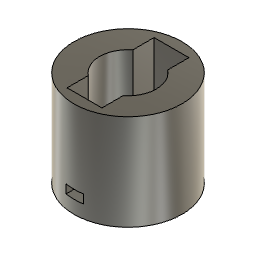
_Button housing.67708ecc-d906-4079-a98f-9e7625d90127 (Autodesk Fusion 360 design; units mm, degrees)
Autodesk Fusion 360 part; units mm, degrees
sketch "Sketch1" plane through (0, 0, 0) normal (0, 0, 1) x (1, 0, 0)
  circle A0 centre (0, 0) radius 31
  dimension "d1" = 62
  constraint coincident A0.centre origin
  measures "d1" diameter of A0
extrude "Extrude1" add sketch "Sketch1" along normal blind 55
sketch "Sketch2" plane through (0, 0, 55) normal (0, 0, 1) x (-1, 0, 0)
  circle A0 centre (0, 0) radius 31
  circle A1 centre (0, 0) radius 16.25
  dimension "d4" = 32.5
  constraint coincident A0.centre A1.centre
  measures "d4" diameter of A1
extrude "Extrude2" cut sketch "Sketch2" against normal blind 50 contours A1
sketch "Sketch3" plane through (0, 0, 55) normal (0, 0, 1) x (-1, 0, 0)
  circle A0 centre (0, 0) radius 16.25
  circle A1 centre (0, 0) radius 31
  line L0 (10, -25) -> (-10, -25)
  line L1 (-10, -25) -> (-10, 25)
  line L2 (-10, 25) -> (10, 25)
  line L3 (10, 25) -> (10, -25)
  line L4 (10, -25) -> (-10, 25) construction
  line L5 (-10, -25) -> (10, 25) construction
  dimension "d7" = 20
  dimension "d8" = 50
  constraint horizontal L0
  constraint perpendicular L0 L1
  constraint parallel L0 L2
  constraint parallel L1 L3
  constraint coincident L4 A0.centre
  constraint coincident L5 A0.centre
  constraint coincident A0.centre A1.centre
  measures "d7" distance of L1.end L2.end
  measures "d8" distance of L0.end L1.end
extrude "Extrude3" cut sketch "Sketch3" against normal blind 50 contours A0 L1 L2 L3 | A0 L0 L1 L3
sketch "Sketch4" plane through (0, -25, 0) normal (0, 1, 0) x (-1, 0, 0)
  line L0 (10, 55) -> (-10, 55)
  line L1 (-10, 55) -> (-10, 5)
  line L2 (-10, 5) -> (10, 5)
  line L3 (10, 5) -> (10, 55)
  line L4 (5, 12.5) -> (-5, 12.5)
  line L5 (-5, 12.5) -> (-5, 7.5)
  line L6 (-5, 7.5) -> (5, 7.5)
  line L7 (5, 7.5) -> (5, 12.5)
  line L8 (5, 12.5) -> (-5, 7.5) construction
  line L9 (-5, 12.5) -> (5, 7.5) construction
  point P0 (0, 10)
  dimension "d11" = 10
  dimension "d12" = 5
  constraint horizontal L4
  constraint perpendicular L4 L5
  constraint parallel L4 L6
  constraint parallel L5 L7
  constraint coincident L8 P0
  constraint coincident L9 P0
  measures "d11" distance of L5.end L6.end
  measures "d12" distance of L4.end L5.end
extrude "Extrude4" cut sketch "Sketch4" against normal blind 8 contours L4 L5 L6 L7
